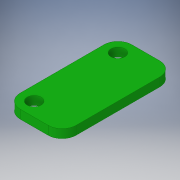
# Autodesk Inventor part: USB_Board
Saved by Autodesk Inventor 2017 (Build 210142000, 142)
## iProperties
Created: 2017-08-03
Part Number: USB_Board
Material: Generic
Document SubType Name: Modeling
Designer: Mitch
Density: 1 g/cm^3
Appearance: Dark Green
Author: Mitch
Autodesk Inventor part; units mm, degrees
ref_plane "YZ Plane" through (0, 0, 0) normal (1, 0, 0) x (0, 1, 0)
ref_plane "XZ Plane" through (0, 0, 0) normal (0, 1, 0) x (-1, 0, 0)
ref_plane "XY Plane" through (0, 0, 0) normal (0, 0, 1) x (1, 0, 0)
sketch "Sketch1" plane through (0, 0, 0) normal (0, 1, 0) x (-1, 0, 0)
  line L0 (2.54, 0) -> (7.62, 0)
  line L1 (10.16, -2.54) -> (10.16, -17.78)
  line L2 (7.62, -20.32) -> (2.54, -20.32)
  line L3 (0, -17.78) -> (0, -2.54)
  arc A0 (10.16, -2.54) -> (7.62, 0) centre (7.62, -2.54) ccw
  arc A1 (7.62, -20.32) -> (10.16, -17.78) centre (7.62, -17.78) ccw
  arc A2 (0, -17.78) -> (2.54, -20.32) centre (2.54, -17.78) ccw
  arc A3 (2.54, 0) -> (0, -2.54) centre (2.54, -2.54) ccw
  circle A4 centre (7.62, -2.54) radius 1.27
  circle A5 centre (7.62, -17.78) radius 1.27
  point P0 (0, 0)
  point P1 (10.16, -20.32)
  point P2 (10.16, 0)
  point P3 (0, -20.32)
  dimension "d0" = 10.16
  dimension "d1" = 20.32
  dimension "d2" = 2.54
  dimension "d3" = 2.54
  dimension "d4" = 2.54
  dimension "d5" = 2.54
  dimension "d6" = 2.54
  dimension "d7" = 2.54
  dimension "d8" = 2.54
  constraints: 8 end point, 8 point on circle, 8 point on line, 8 tangent, 6 centre point, 3 equal radius, 2 parallel, 1 horizontal, 1 perpendicular
  measures "d0" distance of point (10.16, -20.32) point (0, -20.32)
  measures "d1" distance of point (10.16, 0) point (10.16, -20.32)
  measures "d2" radius of A0
  measures "d3" diameter of A4
  measures "d4" distance from line of L1 A4.centre
  measures "d5" distance from line of L0 A4.centre
  measures "d6" diameter of A5
  measures "d7" distance from line of L1 A5.centre
  measures "d8" distance from line of L2 A5.centre
extrude "Extrusion1" add sketch "Sketch1" along normal blind 1.5748
body "Solid1"
